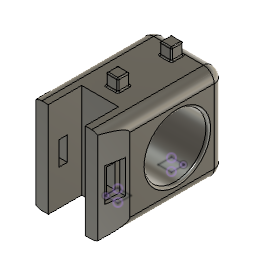
ボンベ固定台_分割式_2026-05-18 (Autodesk Fusion 360 design; units mm, degrees)
Autodesk Fusion 360 part; units mm, degrees
sketch "スケッチ1" plane through (0, 0, 0) normal (0, 0, 1) x (1, 0, 0)
  line L0 (0, 0) -> (-60, 0)
  line L1 (-60, 0) -> (-60, -80)
  line L2 (-60, -80) -> (0, -80)
  line L3 (0, -80) -> (0, 0)
  dimension "d1" = 60
  dimension "d2" = 80
  constraint horizontal L0
  constraint vertical L1
  constraint horizontal L2
  constraint vertical L3
  constraint coincident L0.start L3.end
  measures "d1" distance of L0.start L0.end
  measures "d2" distance of L0.start L2.end
extrude "押し出し1" add sketch "スケッチ1" along normal blind 80
sketch "スケッチ2" plane through (0, 0, 0) normal (1, 0, 0) x (0, 1, 0)
  line L0 (-80, 0) -> (0, 0)
  line L1 (0, 0) -> (0, 80)
  line L2 (0, 80) -> (-80, 80)
  line L3 (-80, 80) -> (-80, 0)
  circle A0 centre (-40, 40) radius 26
  dimension "d5" = 40
  dimension "d6" = 40
  dimension "d7" = 52
  measures "d5" distance of L0 A0.centre
  measures "d6" distance of L1 A0.centre
  measures "d7" diameter of A0
extrude "押し出し2" cut sketch "スケッチ2" against normal blind 60 contours A0
sketch "スケッチ3" plane through (0, 0, 80) normal (0, 0, 1) x (-1, 0, 0)
  line L0 (0, 80) -> (0, 0)
  line L1 (0, 0) -> (60, 0)
  line L2 (60, 0) -> (60, 80)
  line L3 (60, 80) -> (0, 80)
  line L4 (25, 10) -> (35, 10)
  line L5 (35, 10) -> (35, 20)
  line L6 (35, 20) -> (25, 20)
  line L7 (25, 20) -> (25, 10)
  line L8 (25, 55) -> (35, 55)
  line L9 (35, 55) -> (35, 65)
  line L10 (35, 65) -> (25, 65)
  line L11 (25, 65) -> (25, 55)
  dimension "d10" = 10
  dimension "d11" = 25
  dimension "d12" = 25
  dimension "d13" = 15
  dimension "d14" = 10
  dimension "d15" = 10
  dimension "d16" = 10
  dimension "d17" = 10
  constraint horizontal L4
  constraint vertical L5
  constraint horizontal L6
  constraint vertical L7
  constraint horizontal L8
  constraint vertical L9
  constraint horizontal L10
  constraint vertical L11
  measures "d10" distance of L1 L4
  measures "d11" distance of L0 L7
  measures "d12" distance of L0 L11
  measures "d13" distance of L3 L10
  measures "d14" distance of L4 L6
  measures "d15" distance of L8 L10
  measures "d16" distance of L5 L7
  measures "d17" distance of L9 L11
extrude "押し出し3" add sketch "スケッチ3" along normal blind 10 contours L4 L5 L6 L7 | L8 L9 L10 L11
fillet "フィレット1" radius 1 4 faces at (-28.3333, -10, 83.3333) (-25, -16.6667, 83.3333) (-35, -13.3333, 83.3333) (-31.6667, -20, 83.3333)
fillet "フィレット2" radius 1 4 faces at (-35, -58.3333, 83.3333) (-31.6667, -65, 83.3333) (-25, -61.6667, 83.3333) (-28.3333, -55, 83.3333)
extrude "押し出し4" cut sketch "スケッチ3" along normal blind 10 from surface at -80 contours L4 L5 L6 L7 | L8 L9 L10 L11
sketch "スケッチ4" plane through (0, 0, 0) normal (0, 0, 1) x (1, 0, 0)
  line L0 (-45.5, -75) -> (-14.5, -75)
  line L1 (-14.5, -75) -> (-14.5, -106)
  line L2 (-14.5, -106) -> (-45.5, -106)
  line L3 (-45.5, -106) -> (-45.5, -75)
  line L4 (-60, 0) -> (-60, -80)
  line L5 (-60, -80) -> (0, -80)
  dimension "d27" = 14.5
  dimension "d28" = 31
  dimension "d29" = 5
  dimension "d30" = 31
  constraint horizontal L0
  constraint vertical L1
  constraint horizontal L2
  constraint vertical L3
  measures "d27" distance of L0.start L4
  measures "d28" distance of L1.end L2.end
  measures "d29" distance of L0 L5
  measures "d30" distance of L0 L2
sketch "スケッチ5" plane through (0, 0, 0) normal (0, 0, 1) x (1, 0, 0)
  line L0 (-14.5, -106) -> (-45.5, -106)
  line L1 (-45.5, -106) -> (-55.5, -106)
  line L2 (-55.5, -106) -> (-60, -80)
  line L3 (-60, -80) -> (0, -80)
  line L4 (0, -80) -> (-4.5, -106)
  line L5 (-4.5, -106) -> (-14.5, -106)
  dimension "d48" = 26
  dimension "d49" = 10
  dimension "d50" = 10
  dimension "d51" = 4.5
  dimension "d52" = 4.5
  constraint coincident L0.end L1.start
  constraint parallel L0 L1
  constraint parallel L1 L3
  constraint coincident L0.start L5.end
  constraint parallel L0 L5
  measures "d48" distance of L1 L3
  measures "d49" distance of L0.end L1.end
  measures "d50" distance of L4.end L0.start
  measures "d51" horizontal distance of L1.end L2.end
  measures "d52" horizontal distance of L3.end L4.end
extrude "押し出し5" add sketch "スケッチ5" along normal blind 80
extrude "押し出し6" cut sketch "スケッチ4" along normal blind 80
sketch "スケッチ6" plane through (-45.5, 0, 0) normal (1, 0, 0) x (0, 1, 0)
  line L0 (-106, 0) -> (-75, 0)
  line L1 (-75, 0) -> (-75, 80)
  line L2 (-75, 80) -> (-106, 80)
  line L3 (-94, 50) -> (-87, 50)
  line L4 (-87, 50) -> (-87, 30)
  line L5 (-87, 30) -> (-94, 30)
  line L6 (-94, 30) -> (-94, 50)
  line L7 (-106, 80) -> (-106, 0)
  line L8 (-98, 54) -> (-83, 54)
  line L9 (-83, 54) -> (-83, 26)
  line L10 (-83, 26) -> (-98, 26)
  line L11 (-98, 26) -> (-98, 54)
  dimension "d42" = 30
  dimension "d43" = 20
  dimension "d44" = 12
  dimension "d45" = 7
  dimension "d59" = 4
  dimension "d60" = 4
  dimension "d61" = 4
  dimension "d62" = 4
  constraint horizontal L3
  constraint vertical L4
  constraint horizontal L5
  constraint vertical L6
  constraint horizontal L8
  constraint vertical L9
  constraint horizontal L10
  constraint vertical L11
  measures "d42" distance of L2 L3
  measures "d43" distance of L3.start L5.end
  measures "d44" distance of L1 L4
  measures "d45" distance of L3.start L3.end
  measures "d59" distance of L3.start L11
  measures "d60" distance of L4 L9
  measures "d61" distance of L3 L8
  measures "d62" distance of L5 L10
extrude "押し出し7" cut sketch "スケッチ6" along normal mid plane 100 contours L3 L4 L5 L6
fillet "フィレット5" radius 2 1 faces at (-40, -14.1292, 37.4112)
extrude "押し出し8" cut sketch "スケッチ6" along normal blind 5 from surface at 41 contours L8 L9 L10 L11
extrude "押し出し9" cut sketch "スケッチ6" along normal blind 5 from surface at -15 contours L8 L9 L10 L11
fillet "フィレット7" radius 9 4 edges at (-60, -40, 80) (-60, -40, 0) (0, -40, 0) (0, -40, 80) 1 faces at (-20, 0, 26.6667)
sketch "スケッチ7" plane through (0, 0, 0) normal (0, 0, 1) x (1, 0, 0)
  line L0 (-35.5, -65.5) -> (-24.5, -65.5)
  line L1 (-24.5, -65.5) -> (-24.5, -54.5)
  line L2 (-24.5, -54.5) -> (-35.5, -54.5)
  line L3 (-35.5, -54.5) -> (-35.5, -65.5)
  line L4 (-35, -55) -> (-35, -65)
  line L5 (-35, -65) -> (-25, -65)
  line L6 (-24.5, -9.5) -> (-35.5, -9.5)
  line L7 (-35.5, -9.5) -> (-35.5, -20.5)
  line L8 (-35.5, -20.5) -> (-24.5, -20.5)
  line L9 (-24.5, -20.5) -> (-24.5, -9.5)
  line L10 (-25, -10) -> (-35, -10)
  line L11 (-25, -20) -> (-25, -10)
  dimension "d73" = 0.5
  dimension "d74" = 11
  dimension "d75" = 0.5
  dimension "d76" = 11
  dimension "d77" = 0.5
  dimension "d78" = 0.5
  dimension "d79" = 11
  dimension "d80" = 11
  constraint horizontal L0
  constraint vertical L1
  constraint horizontal L2
  constraint vertical L3
  constraint horizontal L6
  constraint vertical L7
  constraint horizontal L8
  constraint vertical L9
  measures "d73" distance of L3 L4
  measures "d74" distance of L0.start L0.end
  measures "d75" distance of L0 L5
  measures "d76" distance of L0.end L1.end
  measures "d77" distance of L6 L10
  measures "d78" distance of L9 L11
  measures "d79" distance of L6.start L6.end
  measures "d80" distance of L6.start L8.end
extrude "押し出し10" cut sketch "スケッチ7" along normal blind 11 contours L0 L1 L2 L3
extrude "押し出し11" cut sketch "スケッチ7" along normal blind 11 contours L6 L7 L8 L9
extrude "押し出し12" cut 1 faces at (-4.5, -84.3333, 36.6667) along direction (-1, 0, 0) blind 1
extrude "押し出し13" cut 1 faces at (-55.5, -84.3333, 36.6667) along direction (1, 0, 0) blind 1
extrude "押し出し14" cut 2 faces at (-11.1667, -106, 52.9317) (-48.8333, -106, 27.0683) along direction (0, 1, 0) blind 2
extrude "押し出し15" cut 1 faces at (-4.5, -105.3333, 27.0683) along direction (1, 0, 0) blind 2
extrude "押し出し16" cut 1 faces at (-55.5, -105.3333, 27.0683) along direction (-1, 0, 0) blind 2
extrude "押し出し17" cut 2 faces at (-11.0513, -104, 27.1384) (-48.9487, -104, 27.1384) along direction (0, 1, 0) blind 1
extrude "押し出し18" cut 1 faces at (-4.1538, -103.3333, 52.8616) along direction (1, 0, 0) blind 2
extrude "押し出し19" cut 1 faces at (-55.8462, -103.3333, 52.8616) along direction (-1, 0, 0) blind 2
